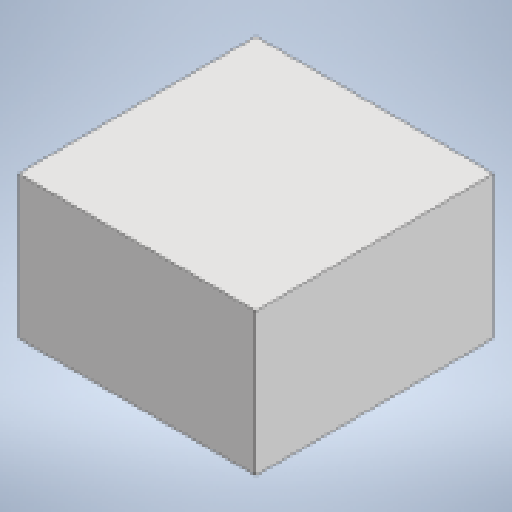
# Autodesk Inventor part: box-1
Saved by Autodesk Inventor 2025 (Build 290162000, 162)
## iProperties
Created: 2026-01-27
Part Number: box-1
Material: 一般
Document SubType Name: Modeling
Designer: mahhy
Density: 1 g/cm^3
Appearance: 既定
Author: mahhy
Autodesk Inventor part; units mm, degrees
ref_plane "YZ Plane" through (0, 0, 0) normal (1, 0, 0) x (0, 1, 0)
ref_plane "XZ Plane" through (0, 0, 0) normal (0, 1, 0) x (-1, 0, 0)
ref_plane "XY Plane" through (0, 0, 0) normal (0, 0, 1) x (1, 0, 0)
sketch "スケッチ1" plane through (0, 0, 0) normal (0, 1, 0) x (-1, 0, 0)
  line L0 (0, 0) -> (-40, 0)
  line L1 (-40, 0) -> (-40, -40)
  line L2 (-40, -40) -> (0, -40)
  line L3 (0, -40) -> (0, 0)
  dimension "d2" = 40
  dimension "d3" = 40
  constraints: 8 end point, 2 parallel, 1 horizontal, 1 perpendicular
  measures "d2" distance of L2.end L1.end
  measures "d3" distance of L1.end L0.end
extrude "押し出し1" add sketch "スケッチ1" along normal blind 17.5
sketch "スケッチ2" plane through (0, 17.5, 0) normal (0, 1, 0) x (1, 0, 0)
  line L0 (2.5, 2.5) -> (37.5, 2.5)
  line L1 (37.5, 2.5) -> (37.5, 37.5)
  line L2 (37.5, 37.5) -> (2.5, 37.5)
  line L3 (2.5, 37.5) -> (2.5, 2.5)
  line L4 (0, 40) -> (0, 0) projected
  line L5 (0, 0) -> (40, 0) projected
  line L6 (40, 40) -> (0, 40) projected
  line L7 (40, 0) -> (40, 40) projected
  dimension "d6" = 2.5
  dimension "d7" = 2.5
  dimension "d8" = 2.5
  dimension "d9" = 2.5
  constraints: 8 end point, 2 parallel, 1 horizontal, 1 perpendicular
  measures "d6" distance between parallel lines of L4 L3
  measures "d7" distance between parallel lines of L5 L0
  measures "d8" distance between parallel lines of L6 L2
  measures "d9" distance between parallel lines of L7 L1
extrude "押し出し2" cut sketch "スケッチ2" against normal blind 12.5 contours L3 L2 L1 L0
equation "\"d3\" = d2"
equation "\"d7\" = d6"
equation "\"d8\" = d6"
equation "\"d9\" = d6"
